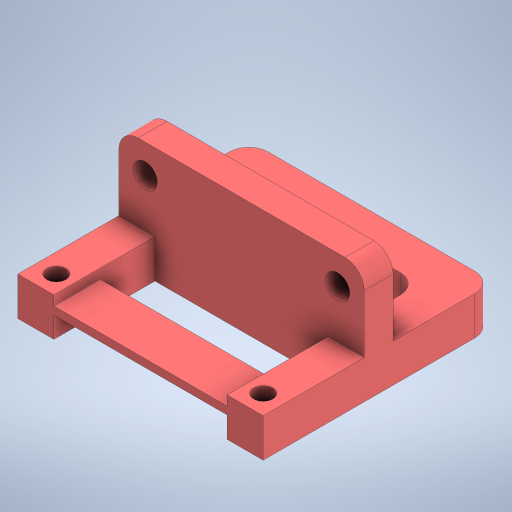
# Autodesk Inventor part: 라즈베리파이 카메라 고정대
Saved by Autodesk Inventor 2023 (Build 270158000, 158)
## iProperties
Created: 2022-08-24
Part Number: 라즈베리파이 카메라 고정대
Material: 일반
Document SubType Name: Modeling
Designer: user
Density: 1 g/cm^3
Appearance: 기본값
Author: user
Autodesk Inventor part; units mm, degrees
ref_plane "YZ Plane" through (0, 0, 0) normal (1, 0, 0) x (0, 1, 0)
ref_plane "XZ Plane" through (0, 0, 0) normal (0, 1, 0) x (-1, 0, 0)
sketch "스케치1" plane through (0, 0, 0) normal (0, 1, 0) x (-1, 0, 0)
  line L0 (-12.75, 12) -> (12.75, 12)
  line L1 (12.75, 12) -> (12.75, -12)
  line L2 (12.75, -12) -> (-12.75, -12)
  line L3 (-12.75, -12) -> (-12.75, 12)
  line L4 (-12.75, 12) -> (12.75, -12) construction
  line L5 (12.75, 12) -> (-12.75, -12) construction
  circle A0 centre (10.75, 10) radius 1
  line L6 (0, 0) -> (3.3414, 0) construction
  line L7 (0, 0) -> (0, -2.4449) construction
  circle A1 centre (-10.75, 10) radius 1
  line L8 (-9, -8) -> (9, -8)
  line L9 (9, -8) -> (9, 12)
  line L10 (9, 12) -> (-9, 12)
  line L11 (-9, 12) -> (-9, -8)
  line L12 (-9, -8) -> (9, 12) construction
  line L13 (9, -8) -> (-9, 12) construction
  circle A2 centre (10.75, -2) radius 1
  circle A3 centre (-10.75, -2) radius 1
  point P0 (0, 2)
  dimension "d0" = 2
  dimension "d1" = 25.5
  dimension "d2" = 24
  dimension "d3" = 2
  dimension "d4" = 2
  dimension "d5" = 18
  dimension "d6" = 20
  dimension "d14" = 12
  constraints: 28 end point, 4 centre point, 4 midpoint, 4 parallel, 3 horizontal, 2 perpendicular, 2 vertical, 1 point on line, 1 symmetric about line, 1 vertical alignment, 5 other
  measures "d0" distance from line of L0 A0.centre
  measures "d1" distance of L0.start L0.end
  measures "d2" distance of L0.end L1.end
  measures "d3" distance from line of L1 A0.centre
  measures "d4" diameter of A0
  measures "d5" distance between parallel lines of L11 L9
  measures "d6" distance of L8.end L9.end
  measures "d14" distance of A0.centre A2.centre
extrude "돌출1" add sketch "스케치1" along normal blind 5 contours L0 L11 L8 L9 L1 L2 L3
sketch "스케치2" plane through (0, 5, 0) normal (0, 1, 0) x (1, 0, 0)
  line L0 (-9, -12) -> (-9, 8) projected
  line L1 (9, 1.5) -> (-9, 1.5)
  line L2 (-9, 1.5) -> (-9, -1.5)
  line L3 (-9, -1.5) -> (9, -1.5)
  line L4 (9, -1.5) -> (9, 1.5)
  line L5 (9, 1.5) -> (-9, -1.5) construction
  line L6 (-9, 1.5) -> (9, -1.5) construction
  line L7 (-12.75, -12) -> (-9, -12) projected
  line L8 (-12.75, 12) -> (-12.75, -12) projected
  line L9 (-9, 1.5) -> (-12.75, 1.5)
  line L10 (-12.75, 1.5) -> (-12.75, -1.5)
  line L11 (-12.75, -1.5) -> (-9, -1.5)
  line L12 (-9, -1.5) -> (-9, 1.5)
  line L13 (12.75, -12) -> (12.75, 12) projected
  line L14 (9, 1.5) -> (12.75, 1.5)
  line L15 (12.75, 1.5) -> (12.75, -1.5)
  line L16 (12.75, -1.5) -> (9, -1.5)
  line L17 (9, -1.5) -> (9, 1.5)
  point P0 (0, 0)
  point P1 (0, 0)
  point P2 (-9, 1.5)
  point P3 (-9, 1.5)
  dimension "d16" = 10.5
  dimension "d17" = 3
  constraints: 28 end point, 6 parallel, 4 point on line, 3 horizontal, 3 perpendicular, 2 midpoint
  measures "d16" distance between parallel lines of L7 L3
  measures "d17" distance of L1.end L2.end
extrude "돌출2" add sketch "스케치2" along normal blind 7 and the other way blind 5 contours L11 L8 L9 L0 | L0 L1 L4 L3 | L4 L14 L13 L16
fillet "모깎기1" radius 2 4 edges at (-9, 2.5, -8) (9, 2.5, -8) (-12.75, 2.5, -12) (12.75, 2.5, -12)
fillet "모깎기4" radius 2 2 edges at (-12.75, 12, 0) (12.75, 12, 0)
ref_plane "작업 평면1" through (0, 2.2, 0) normal (0, -1, 0) x (1, 0, 0)
sketch "스케치5" plane through (0, 2.2, 0) normal (0, -1, 0) x (1, 0, 0)
  line L0 (-12.75, 12) -> (-9, 12) projected
  line L1 (9, 1.5) -> (9, 12) projected
  line L2 (-9, 12) -> (9, 12)
  line L3 (9, 12) -> (9, 7)
  line L4 (9, 7) -> (-9, 7)
  line L5 (-9, 7) -> (-9, 12)
  point P0 (0, 0)
  point P1 (9, 3.5)
  point P2 (-11.25, 12)
  dimension "d43" = 5
  constraints: 8 end point, 2 parallel, 1 horizontal, 1 perpendicular, 1 point on line
  measures "d43" distance between parallel lines of L2 L4
extrude "돌출5" add sketch "스케치5" against normal up to surface (2.8 mm away)
chamfer "모따기1" distance 1 angle 45 1 edges at (0, 2.2, 7)
sketch "스케치6" plane through (0, 5, 0) normal (0, 1, 0) x (1, 0, 0)
  line L0 (-9, -7) -> (9, -7) projected
  line L1 (-12.75, -12) -> (12.75, -12) projected
  line L2 (-9, -7) -> (9, -7)
  line L3 (9, -7) -> (9, -12)
  line L4 (9, -12) -> (-9, -12)
  line L5 (-9, -12) -> (-9, -7)
  point P0 (0, 0)
  point P1 (-9, -12)
  point P2 (-11.25, -12)
  point P3 (11.25, -12)
  point P4 (10.5, -12)
  constraints: 8 end point, 2 parallel, 1 horizontal, 1 perpendicular, 1 point on line
extrude "돌출6" cut sketch "스케치6" against normal blind 2
extrude "돌출7" cut sketch "스케치1" along normal blind 5 contours A2 | A3
sketch "스케치8" plane through (-12.75, 5, 1.5) normal (0, 0, 1) x (1, 0, 0)
  circle A0 centre (2.75, 4) radius 1.25
  line L0 (21.75, -5) -> (3.75, -5) projected
  line L1 (12.75, -5) -> (12.75, 3.7696)
  circle A1 centre (22.75, 4) radius 1.25
  line L2 (2, 7) -> (23.5, 7) projected
  point P0 (12.75, -5)
  dimension "d53" = 2.5
  dimension "d54" = 10
  dimension "d55" = 3
  constraints: 2 centre point, 2 end point, 1 midpoint, 1 symmetric about line, 1 vertical, 1 other
  measures "d53" diameter of A0
  measures "d54" horizontal distance of L1.start A0.centre
  measures "d55" distance from line of L2 A0.centre
extrude "돌출8" cut sketch "스케치8" against normal blind 5
sketch "스케치10" plane through (0, 5, 0) normal (0, 1, 0) x (1, 0, 0)
  line L0 (9, -1.5) -> (9, -12) projected
  line L1 (9, -12) -> (12.75, -12) projected
  line L2 (12.75, -12) -> (12.75, -1.5) projected
  line L3 (12.75, -1.5) -> (9, -1.5) projected
  circle A0 centre (10.75, -10) radius 1 projected
  line L4 (-9, -12) -> (-9, -1.5) projected
  line L5 (-9, -1.5) -> (-12.75, -1.5) projected
  line L6 (-12.75, -1.5) -> (-12.75, -12) projected
  line L7 (-12.75, -12) -> (-9, -12) projected
  circle A1 centre (-10.75, -10) radius 1 projected
  arc A2 (12.75, 10) -> (10.75, 12) centre (10.75, 10) ccw projected
  line L8 (10.75, 12) -> (-10.75, 12) projected
  arc A3 (-10.75, 12) -> (-12.75, 10) centre (-10.75, 10) ccw projected
  line L9 (-12.75, 10) -> (-12.75, 1.5) projected
  line L10 (-12.75, 1.5) -> (-11.616, 1.5) projected
  arc A4 (-9.884, 1.5) -> (-11.616, 1.5) centre (-10.75, 2) ccw projected
  line L11 (-9.884, 1.5) -> (-9, 1.5) projected
  line L12 (-9, 1.5) -> (-9, 6) projected
  arc A5 (-7, 8) -> (-9, 6) centre (-7, 6) ccw projected
  line L13 (-7, 8) -> (7, 8) projected
  arc A6 (9, 6) -> (7, 8) centre (7, 6) ccw projected
  line L14 (9, 6) -> (9, 1.5) projected
  line L15 (9, 1.5) -> (9.884, 1.5) projected
  arc A7 (11.616, 1.5) -> (9.884, 1.5) centre (10.75, 2) ccw projected
  line L16 (11.616, 1.5) -> (12.75, 1.5) projected
  line L17 (12.75, 1.5) -> (12.75, 10) projected
  point P0 (0, 0)
extrude "돌출10" cut sketch "스케치10" against normal blind 1
